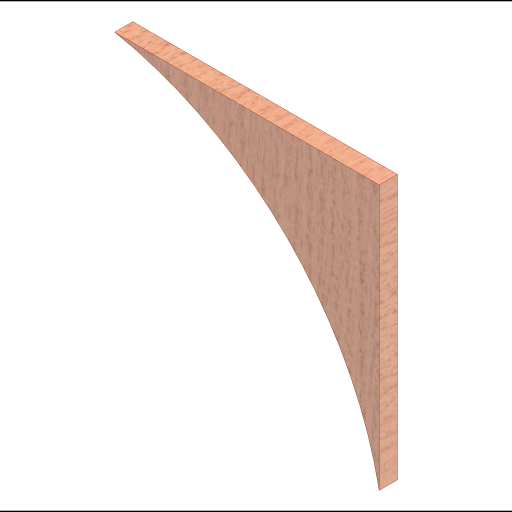
# Autodesk Inventor part: Wind Tunnel Fan Shroud Corner
Saved by Autodesk Inventor 2023 (Build 270158000, 158)
## iProperties
Created: 2022-01-23
Part Number: Wind Tunnel Fan Shroud Corner
Material: Wood (Oak)
Document SubType Name: Modeling
Designer: kamer
Density: 0.76 g/cm^3
Appearance: White Oak - Natural Medium Gloss
Author: kamer
Autodesk Inventor part; units mm, degrees
ref_plane "YZ Plane" through (0, 0, 0) normal (1, 0, 0) x (0, 1, 0)
ref_plane "XZ Plane" through (0, 0, 0) normal (0, 1, 0) x (-1, 0, 0)
ref_plane "XY Plane" through (0, 0, 0) normal (0, 0, 1) x (1, 0, 0)
sketch "Sketch1" plane through (0, 0, 0) normal (0, 0, 1) x (1, 0, 0)
  circle A0 centre (0, 0) radius 215.9
  line L0 (-215.9, 215.9) -> (215.9, 215.9)
  line L1 (215.9, 215.9) -> (215.9, -215.9)
  line L2 (215.9, -215.9) -> (-215.9, -215.9)
  line L3 (-215.9, -215.9) -> (-215.9, 215.9)
  point P0 (215.9, 0)
  point P1 (0, 215.9)
  dimension "d0" = 431.8
  dimension "d1" = 431.8
  dimension "d2" = 431.8
  dimension "d3" = 215.9
  dimension "d4" = 215.9
  constraints: 8 end point, 2 parallel, 1 centre point, 1 coincident, 1 horizontal, 1 perpendicular
  measures "d0" diameter of A0
  measures "d1" distance of L1.end L2.end
  measures "d2" distance of L0.end L1.end
  measures "d3" distance from line of L3 point (0, 0)
  measures "d4" distance from line of L0 point (0, 0)
extrude "Extrusion1" add sketch "Sketch1" along normal blind 11.938 contours A0 L0 L1
sketch "Sketch2" plane through (0, 0, 11.938) normal (0, 0, 1) x (1, 0, 0)
  circle A0 centre (0, 0) radius 220
  dimension "d7" = 440
  constraints: 1 centre point, 1 coincident
  measures "d7" diameter of A0
extrude "Extrusion2" cut sketch "Sketch2" against normal through all
body "Solid1"
